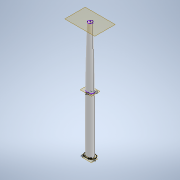
# Autodesk Inventor part: fuselage
Saved by Autodesk Inventor 2022 (Build 260153000, 153)
## iProperties
Created: 2021-03-11
Part Number: fuselage
Material: Generic
Document SubType Name: Modeling
Designer: Ferdinand Hubbard
Density: 1 g/cm^3
Appearance: Default
Author: Ferdinand Hubbard
Autodesk Inventor part; units mm, degrees
ref_plane "YZ Plane" through (0, 0, 0) normal (1, 0, 0) x (0, 1, 0)
ref_plane "XY Plane" through (0, 0, 0) normal (0, 0, 1) x (1, 0, 0)
sketch "Sketch1" plane through (0, 0, 0) normal (0, 1, 0) x (-1, 0, 0)
  ellipse E0 centre (0, 0) end of major axis (31, 0) minor radius 21
  dimension "d8" = 21
  dimension "d9" = 31
  constraints: 1 centre point
ref_plane "Work Plane1" through (0, 463, 0) normal (0, 1, 0) x (-1, 0, 0)
sketch "Sketch2" plane through (0, 463, 0) normal (0, 1, 0) x (-1, 0, 0)
  circle A0 centre (0, 0) radius 16
  dimension "d57" = 32
  constraints: 1 centre point
  measures "d57" diameter of A0
sketch "Sketch3" plane through (0, 463, 0) normal (0, 1, 0) x (-1, 0, 0)
  circle A0 centre (0, 0) radius 16.5
  dimension "d58" = 33
  constraints: 1 centre point
  measures "d58" diameter of A0
sketch "Sketch4" plane through (0, 0, 0) normal (0, 1, 0) x (-1, 0, 0)
  ellipse E0 centre (0, 0) end of major axis (0, 20) minor radius 30
  dimension "d19" = 20
  dimension "d20" = 30
  constraints: 1 coincident, 2 other
ref_plane "Work Plane3" through (0, -435, 0) normal (0, 1, 0) x (-1, 0, 0)
ref_plane "Work Plane2" through (0, -455, 0) normal (0, 1, 0) x (-1, 0, 0)
sketch "Sketch5" plane through (0, -435, 0) normal (0, 1, 0) x (-1, 0, 0)
  ellipse E0 centre (0, 0) end of major axis (-31, 0) minor radius 21
  dimension "d27" = 21
  dimension "d28" = 31
  constraints: 1 coincident, 2 other
sketch "Sketch6" plane through (0, -435, 0) normal (0, 1, 0) x (-1, 0, 0)
  ellipse E0 centre (0, 0) end of major axis (-40, 0) minor radius 30
  dimension "d29" = 40
  dimension "d30" = 30
  constraints: 1 coincident, 2 other
sketch "Sketch7" plane through (0, -455, 0) normal (0, 1, 0) x (-1, 0, 0)
  circle A0 centre (0, 0) radius 5
  dimension "d31" = 10
  constraints: 1 centre point, 1 coincident
  measures "d31" diameter of A0
sketch "Sketch8" plane through (0, -455, 0) normal (0, 1, 0) x (-1, 0, 0)
  circle A0 centre (0, 0) radius 6
  dimension "d32" = 12
  constraints: 1 centre point, 1 coincident
  measures "d32" diameter of A0
loft "Loft9" add profiles "Sketch3", "Sketch1", "Sketch5"
body "Solid3"
